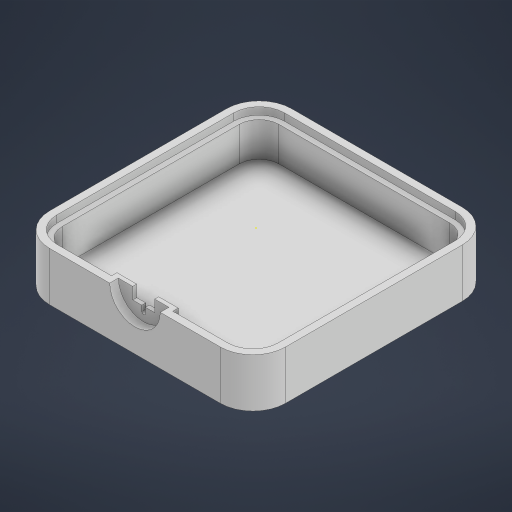
# Autodesk Inventor part: enclosure_i
Saved by Autodesk Inventor 2024 (Build 280153000, 153)
## iProperties
Created: 2023-07-19
Part Number: enclosure_i
Material: Generic
Document SubType Name: Modeling
Designer: LabTel_Admin
Density: 1 g/cm^3
Appearance: Default
Author: LabTel_Admin
Autodesk Inventor part; units mm, degrees
ref_plane "YZ Plane" through (0, 0, 0) normal (1, 0, 0) x (0, 1, 0)
ref_plane "XZ Plane" through (0, 0, 0) normal (0, 1, 0) x (-1, 0, 0)
sketch "Sketch1" plane through (0, 0, 0) normal (0, 1, 0) x (-1, 0, 0)
  line L0 (-23.65, -33.5) -> (23.65, -33.5)
  line L1 (32.65, -24.5) -> (32.65, 24.5)
  line L2 (23.65, 33.5) -> (-23.65, 33.5)
  line L3 (-32.65, 24.5) -> (-32.65, -24.5)
  line L4 (-32.65, -33.5) -> (32.65, 33.5) construction
  line L5 (32.65, -33.5) -> (-32.65, 33.5) construction
  arc A0 (32.65, 24.5) -> (23.65, 33.5) centre (23.65, 24.5) ccw
  arc A1 (23.65, -33.5) -> (32.65, -24.5) centre (23.65, -24.5) ccw
  arc A2 (-32.65, -24.5) -> (-23.65, -33.5) centre (-23.65, -24.5) ccw
  arc A3 (-23.65, 33.5) -> (-32.65, 24.5) centre (-23.65, 24.5) ccw
  line L6 (29.15, 24.5) -> (29.15, -24.5)
  arc A4 (23.65, -30) -> (29.15, -24.5) centre (23.65, -24.5) ccw
  line L7 (23.65, -30) -> (-23.65, -30)
  arc A5 (-29.15, -24.5) -> (-23.65, -30) centre (-23.65, -24.5) ccw
  line L8 (-29.15, -24.5) -> (-29.15, 24.5)
  arc A6 (-23.65, 30) -> (-29.15, 24.5) centre (-23.65, 24.5) ccw
  line L9 (-23.65, 30) -> (23.65, 30)
  arc A7 (29.15, 24.5) -> (23.65, 30) centre (23.65, 24.5) ccw
  line L10 (23.65, -32) -> (-23.65, -32)
  arc A8 (-31.15, -24.5) -> (-23.65, -32) centre (-23.65, -24.5) ccw
  line L11 (-31.15, -24.5) -> (-31.15, 24.5)
  arc A9 (-23.65, 32) -> (-31.15, 24.5) centre (-23.65, 24.5) ccw
  line L12 (-23.65, 32) -> (23.65, 32)
  arc A10 (31.15, 24.5) -> (23.65, 32) centre (23.65, 24.5) ccw
  line L13 (31.15, 24.5) -> (31.15, -24.5)
  arc A11 (23.65, -32) -> (31.15, -24.5) centre (23.65, -24.5) ccw
  point P0 (0, 0)
  point P1 (32.65, 0)
  point P2 (31.5, 26.5247)
  dimension "d3" = 9
  dimension "d4" = 9
  dimension "d5" = 3.5
  dimension "d44" = 1.5
  dimension "d72" = 58.3
  dimension "d73" = 60
  constraints: 28 end point, 24 point on circle, 12 centre point, 8 point on line, 8 tangent, 6 parallel, 3 midpoint, 3 perpendicular, 2 equal radius, 1 horizontal, 14 other
  measures "d3" radius of A0
  measures "d4" radius of A1
  measures "d5" distance between parallel lines of L1 L6
  measures "d44" distance between parallel lines of L0 L10
  measures "d72" distance between parallel lines of L8 L6
  measures "d73" distance between parallel lines of L9 L7
extrude "Extrusion1" add sketch "Sketch1" along normal blind 2 contours L6 A4 L7 A5 L8 A6 L9 A7
extrude "Extrusion2" add sketch "Sketch1" along normal blind 13.5 contours A2 L3 A3 L2 A0 L1 A1 L0 | L10 A8 L11 A9 L12 A10 L13 A11
sketch "Sketch2" plane through (-23.65, 0, 33.5) normal (0, 0, 1) x (1, 0, 0)
  line L0 (0, 13.5) -> (47.3, 13.5) projected
  arc A0 (16.65, 13.5) -> (30.65, 13.5) centre (23.65, 13.5) ccw
  line L1 (16.65, 13.5) -> (30.65, 13.5)
  point P0 (23.65, 0)
  dimension "d10" = 14
  constraints: 2 end point, 2 point on circle, 2 point on line, 1 centre point, 1 collinear, 1 midpoint
  measures "d10" diameter of A0
extrude "Extrusion3" cut sketch "Sketch2" against normal blind 2.4
sketch "Sketch3" plane through (-23.65, 0, 31.1) normal (0, 0, 1) x (1, 0, 0)
  line L0 (26.7, 10.25) -> (20.6, 10.25)
  line L1 (20.6, 10.25) -> (20.6, 13.5)
  line L2 (26.7, 13.5) -> (26.7, 10.25)
  line L3 (16.65, 13.5) -> (30.65, 13.5) projected
  line L4 (26.7, 10.25) -> (23.65, 13.5) construction
  line L5 (20.6, 10.25) -> (26.7, 16.75) construction
  line L6 (20.6, 13.5) -> (26.7, 13.5)
  line L7 (24.15, 10.25) -> (24.15, 8.75)
  line L8 (23.65, 8.25) -> (23.65, 8.25)
  line L9 (23.15, 8.75) -> (23.15, 10.25)
  line L10 (23.65, 10.25) -> (24.15, 8.25) construction
  line L11 (23.65, 10.25) -> (23.15, 8.25) construction
  arc A0 (23.65, 8.25) -> (24.15, 8.75) centre (23.65, 8.75) ccw
  arc A1 (23.15, 8.75) -> (23.65, 8.25) centre (23.65, 8.75) ccw
  point P0 (23.65, 0)
  point P1 (23.65, 8.25)
  dimension "d13" = 6.5
  dimension "d15" = 1
  dimension "d17" = 0.5
  dimension "d75" = 6.1
  constraints: 22 end point, 8 point on line, 5 midpoint, 4 point on circle, 4 tangent, 2 centre point, 2 parallel, 1 concentric, 1 horizontal, 1 perpendicular
  measures "d13" distance of L5.end L0.start
  measures "d15" distance of L10.end L11.end
  measures "d17" radius of A0
  measures "d75" distance between parallel lines of L2 L1
extrude "Extrusion4" cut sketch "Sketch3" against normal blind 2
ref_plane "Work Plane1" through (0, -1, 0) normal (0, -1, 0) x (1, 0, 0)
sketch "Sketch5" plane through (0, -1, 0) normal (0, -1, 0) x (1, 0, 0)
  line L0 (-30.0692, 3.0119) -> (30.4708, 3.0119) construction
  line L1 (30.4708, 3.0119) -> (30.4708, -30.1194) construction
  line L2 (30.4708, -30.1194) -> (-30.0692, -30.1194) construction
  line L3 (-30.0692, -30.1194) -> (-30.0692, 3.0119) construction
  line L4 (-9.6136, -3.095) -> (-7.5909, 2.905)
  line L5 (-7.5909, 2.905) -> (-6.6088, 2.905)
  line L6 (-6.6088, 2.905) -> (-4.5861, -3.095)
  line L7 (-4.5861, -3.095) -> (-5.4272, -3.095)
  line L8 (-5.4272, -3.095) -> (-5.9718, -1.4176)
  line L9 (-5.9718, -1.4176) -> (-8.2619, -1.4176)
  line L10 (-8.2619, -1.4176) -> (-8.8065, -3.095)
  line L11 (-8.8065, -3.095) -> (-9.6136, -3.095)
  line L12 (-6.1906, -0.7368) -> (-7.1193, 2.0881)
  line L13 (-7.1193, 2.0881) -> (-8.0431, -0.7368)
  line L14 (-8.0431, -0.7368) -> (-6.1906, -0.7368)
  spline S0 degree 2 poles (-2.3446, -3.202) (-2.9961, -3.202) (-3.9102, -2.9297) (-4.3138, -2.7352) knots 0 0 0 1 2 2 2
  line L15 (-4.3138, -2.7352) -> (-4.3138, -1.7336)
  line L16 (-4.3138, -1.7336) -> (-4.2554, -1.7336)
  spline S1 degree 2 poles (-4.2554, -1.7336) (-3.8616, -2.1031) (-2.8648, -2.5116) (-2.4029, -2.5116) knots 0 0 0 1 2 2 2
  spline S2 degree 2 poles (-2.4029, -2.5116) (-1.7417, -2.5116) (-1.0658, -1.9621) (-1.0658, -1.5099) knots 0 0 0 1 2 2 2
  spline S3 degree 2 poles (-1.0658, -1.5099) (-1.0658, -1.1501) (-1.4208, -0.7028) (-1.8049, -0.591) knots 0 0 0 1 2 2 2
  spline S4 degree 2 poles (-1.8049, -0.591) (-2.082, -0.5132) (-2.5439, -0.4062) (-2.8892, -0.3187) knots 0 0 0 1 2 2 2
  spline S5 degree 2 poles (-2.8892, -0.3187) (-3.2003, -0.236) (-3.6914, 0.0119) (-3.8811, 0.2113) knots 0 0 0 1 2 2 2
  spline S6 degree 2 poles (-3.8811, 0.2113) (-4.0658, 0.4106) (-4.27, 0.9455) (-4.27, 1.2956) knots 0 0 0 1 2 2 2
  spline S7 degree 2 poles (-4.27, 1.2956) (-4.27, 2.0249) (-3.1323, 3.0119) (-2.2522, 3.0119) knots 0 0 0 1 2 2 2
  spline S8 degree 2 poles (-2.2522, 3.0119) (-1.7465, 3.0119) (-0.8519, 2.8126) (-0.4678, 2.623) knots 0 0 0 1 2 2 2
  line L17 (-0.4678, 2.623) -> (-0.4678, 1.67)
  line L18 (-0.4678, 1.67) -> (-0.5261, 1.67)
  spline S9 degree 2 poles (-0.5261, 1.67) (-0.813, 1.9325) (-1.7076, 2.3215) (-2.1987, 2.3215) knots 0 0 0 1 2 2 2
  spline S10 degree 2 poles (-2.1987, 2.3215) (-2.753, 2.3215) (-3.4386, 1.8012) (-3.4386, 1.3782) knots 0 0 0 1 2 2 2
  spline S11 degree 2 poles (-3.4386, 1.3782) (-3.4386, 0.999) (-3.035, 0.5468) (-2.6558, 0.4447) knots 0 0 0 1 2 2 2
  spline S12 degree 2 poles (-2.6558, 0.4447) (-2.4029, 0.3766) (-1.6687, 0.2016) (-1.4256, 0.1286) knots 0 0 0 1 2 2 2
  spline S13 degree 2 poles (-1.4256, 0.1286) (-0.8081, -0.061) (-0.2344, -0.8244) (-0.2344, -1.3835) knots 0 0 0 1 2 2 2
  spline S14 degree 2 poles (-0.2344, -1.3835) (-0.2344, -1.7385) (-0.5212, -2.4192) (-0.7789, -2.6574) knots 0 0 0 1 2 2 2
  spline S15 degree 2 poles (-0.7789, -2.6574) (-1.0658, -2.92) (-1.7952, -3.202) (-2.3446, -3.202) knots 0 0 0 1 2 2 2
  spline S16 degree 2 poles (2.6732, -3.2214) (2.1433, -3.2214) (1.3556, -2.9443) (1.0784, -2.6672) knots 0 0 0 1 2 2 2
  spline S17 degree 2 poles (1.0784, -2.6672) (0.7624, -2.356) (0.5047, -1.4808) (0.5047, -0.8389) knots 0 0 0 1 2 2 2
  line L19 (0.5047, -0.8389) -> (0.5047, 2.905)
  line L20 (0.5047, 2.905) -> (1.3021, 2.905)
  line L21 (1.3021, 2.905) -> (1.3021, -0.8389)
  spline S18 degree 2 poles (1.3021, -0.8389) (1.3021, -1.2571) (1.4091, -1.8211) (1.5598, -2.0496) knots 0 0 0 1 2 2 2
  spline S19 degree 2 poles (1.5598, -2.0496) (1.7202, -2.2928) (2.2745, -2.5407) (2.6732, -2.5407) knots 0 0 0 1 2 2 2
  spline S20 degree 2 poles (2.6732, -2.5407) (3.0476, -2.5407) (3.6311, -2.2928) (3.7916, -2.0496) knots 0 0 0 1 2 2 2
  spline S21 degree 2 poles (3.7916, -2.0496) (3.9423, -1.8211) (4.0493, -1.262) (4.0493, -0.8584) knots 0 0 0 1 2 2 2
  line L22 (4.0493, -0.8584) -> (4.0493, 2.905)
  line L23 (4.0493, 2.905) -> (4.8467, 2.905)
  line L24 (4.8467, 2.905) -> (4.8467, -0.8389)
  spline S22 degree 2 poles (4.8467, -0.8389) (4.8467, -1.4662) (4.5938, -2.3608) (4.2729, -2.6672) knots 0 0 0 1 2 2 2
  spline S23 degree 2 poles (4.2729, -2.6672) (3.986, -2.9492) (3.2275, -3.2214) (2.6732, -3.2214) knots 0 0 0 1 2 2 2
  spline S24 degree 2 poles (7.6619, -3.202) (7.0104, -3.202) (6.0963, -2.9297) (5.6927, -2.7352) knots 0 0 0 1 2 2 2
  line L25 (5.6927, -2.7352) -> (5.6927, -1.7336)
  line L26 (5.6927, -1.7336) -> (5.751, -1.7336)
  spline S25 degree 2 poles (5.751, -1.7336) (6.1449, -2.1031) (7.1416, -2.5116) (7.6036, -2.5116) knots 0 0 0 1 2 2 2
  spline S26 degree 2 poles (7.6036, -2.5116) (8.2648, -2.5116) (8.9407, -1.9621) (8.9407, -1.5099) knots 0 0 0 1 2 2 2
  spline S27 degree 2 poles (8.9407, -1.5099) (8.9407, -1.1501) (8.5857, -0.7028) (8.2016, -0.591) knots 0 0 0 1 2 2 2
  spline S28 degree 2 poles (8.2016, -0.591) (7.9245, -0.5132) (7.4625, -0.4062) (7.1173, -0.3187) knots 0 0 0 1 2 2 2
  spline S29 degree 2 poles (7.1173, -0.3187) (6.8061, -0.236) (6.3151, 0.0119) (6.1254, 0.2113) knots 0 0 0 1 2 2 2
  spline S30 degree 2 poles (6.1254, 0.2113) (5.9407, 0.4106) (5.7365, 0.9455) (5.7365, 1.2956) knots 0 0 0 1 2 2 2
  spline S31 degree 2 poles (5.7365, 1.2956) (5.7365, 2.0249) (6.8742, 3.0119) (7.7543, 3.0119) knots 0 0 0 1 2 2 2
  spline S32 degree 2 poles (7.7543, 3.0119) (8.26, 3.0119) (9.1546, 2.8126) (9.5387, 2.623) knots 0 0 0 1 2 2 2
  line L27 (9.5387, 2.623) -> (9.5387, 1.67)
  line L28 (9.5387, 1.67) -> (9.4804, 1.67)
  spline S33 degree 2 poles (9.4804, 1.67) (9.1935, 1.9325) (8.2989, 2.3215) (7.8078, 2.3215) knots 0 0 0 1 2 2 2
  spline S34 degree 2 poles (7.8078, 2.3215) (7.2535, 2.3215) (6.5679, 1.8012) (6.5679, 1.3782) knots 0 0 0 1 2 2 2
  spline S35 degree 2 poles (6.5679, 1.3782) (6.5679, 0.999) (6.9715, 0.5468) (7.3507, 0.4447) knots 0 0 0 1 2 2 2
  spline S36 degree 2 poles (7.3507, 0.4447) (7.6036, 0.3766) (8.3377, 0.2016) (8.5809, 0.1286) knots 0 0 0 1 2 2 2
  spline S37 degree 2 poles (8.5809, 0.1286) (9.1984, -0.061) (9.7721, -0.8244) (9.7721, -1.3835) knots 0 0 0 1 2 2 2
  spline S38 degree 2 poles (9.7721, -1.3835) (9.7721, -1.7385) (9.4852, -2.4192) (9.2275, -2.6574) knots 0 0 0 1 2 2 2
  spline S39 degree 2 poles (9.2275, -2.6574) (8.9407, -2.92) (8.2113, -3.202) (7.6619, -3.202) knots 0 0 0 1 2 2 2
  point P0 (0, 0)
  constraints: 2 other
extrude "Extrusion5" cut sketch "Sketch5" against normal blind 1.2
sketch "Boceto12" plane through (0, 13.5, 0) normal (0, 1, 0) x (1, 0, 0)
  point P0 (0, 0)
sketch "Boceto13" plane through (0, 13.5, 0) normal (0, 1, 0) x (1, 0, 0)
  line L0 (32.65, -24.5) -> (32.65, 24.5) projected
  arc A0 (32.65, 24.5) -> (23.65, 33.5) centre (23.65, 24.5) ccw projected
  line L1 (23.65, 33.5) -> (-23.65, 33.5) projected
  arc A1 (-23.65, 33.5) -> (-32.65, 24.5) centre (-23.65, 24.5) ccw projected
  line L2 (-32.65, 24.5) -> (-32.65, -24.5) projected
  arc A2 (-32.65, -24.5) -> (-23.65, -33.5) centre (-23.65, -24.5) ccw projected
  line L3 (-23.65, -33.5) -> (-7, -33.5) projected
  line L4 (7, -33.5) -> (23.65, -33.5) projected
  arc A3 (23.65, -33.5) -> (32.65, -24.5) centre (23.65, -24.5) ccw projected
  line L5 (-8.5, -31.51) -> (-23.65, -31.51)
  arc A4 (-30.66, -24.5) -> (-23.65, -31.51) centre (-23.65, -24.5) ccw
  line L6 (-30.66, -24.5) -> (-30.66, 24.5)
  arc A5 (-23.65, 31.51) -> (-30.66, 24.5) centre (-23.65, 24.5) ccw
  line L7 (-23.65, 31.51) -> (23.65, 31.51)
  arc A6 (30.66, 24.5) -> (23.65, 31.51) centre (23.65, 24.5) ccw
  line L8 (30.66, 24.5) -> (30.66, -24.5)
  arc A7 (23.65, -31.51) -> (30.66, -24.5) centre (23.65, -24.5) ccw
  line L9 (-23.65, -30) -> (23.65, -30) projected
  arc A8 (23.65, -30) -> (29.15, -24.5) centre (23.65, -24.5) ccw projected
  line L10 (29.15, 24.5) -> (29.15, -24.5) projected
  arc A9 (29.15, 24.5) -> (23.65, 30) centre (23.65, 24.5) ccw projected
  line L11 (-23.65, 30) -> (23.65, 30) projected
  arc A10 (-23.65, 30) -> (-29.15, 24.5) centre (-23.65, 24.5) ccw projected
  line L12 (-29.15, -24.5) -> (-29.15, 24.5) projected
  arc A11 (-29.15, -24.5) -> (-23.65, -30) centre (-23.65, -24.5) ccw projected
  line L13 (-3.05, -30) -> (-23.65, -30) projected
  line L14 (29.15, 24.5) -> (29.15, -24.5)
  line L15 (23.65, -30) -> (8.5, -30)
  line L16 (-8.5, -30) -> (-23.65, -30)
  line L17 (-29.15, -24.5) -> (-29.15, 24.5)
  line L18 (-23.65, 30) -> (23.65, 30)
  arc A12 (29.15, 24.5) -> (23.65, 30) centre (23.65, 24.5) ccw
  arc A13 (23.65, -30) -> (29.15, -24.5) centre (23.65, -24.5) ccw projected
  arc A14 (23.65, -30) -> (29.15, -24.5) centre (23.65, -24.5) ccw
  arc A15 (-29.15, -24.5) -> (-23.65, -30) centre (-23.65, -24.5) ccw
  arc A16 (-23.65, 30) -> (-29.15, 24.5) centre (-23.65, 24.5) ccw
  line L19 (-8.5, -31.51) -> (-8.5, -30)
  line L20 (-7, -33.5) -> (-7, -31.1) projected
  line L21 (7, -31.1) -> (7, -33.5) projected
  line L22 (8.5, -30) -> (8.5, -31.51)
  line L23 (8.5, -31.51) -> (23.65, -31.51)
  point P0 (0, 0)
  point P1 (-8.5, -30)
  point P2 (8.5, -30)
  dimension "d45" = 1.99
  dimension "d48" = 1.5
  dimension "d76" = 1.5
  constraints: 24 end point, 20 point on circle, 8 centre point, 3 concentric, 3 tangent, 2 collinear, 2 perpendicular, 1 point on line, 1 vertical, 6 other
  measures "d45" distance between parallel lines of L0 L8
  measures "d48" distance between parallel lines of L20 L19
  measures "d76" distance between parallel lines of L21 L22
extrude "Extrusión11" cut sketch "Boceto13" against normal blind 2 contours L5 A4 L6 A5 L7 A6 L8 A7 L23 L22 L9 A8 L10 A9 L11 A10 L12 A11 L19
equation "\"andho_sobresalto\" = 5"
body "Solid1"
